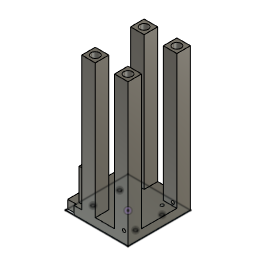
airbee_middle (Autodesk Fusion 360 design; units mm, degrees)
Autodesk Fusion 360 part; units mm, degrees
note: some values were not read from the file. Set by a fixed rule: which sketch regions a step uses.
sketch "Skizze1" plane through (0, 0, 0) normal (0, 0, 1) x (1, 0, 0)
  line L0 (-15.05, 15.05) -> (14.75, 15.05)
  line L1 (14.75, 15.05) -> (14.75, -14.75)
  line L2 (14.75, -14.75) -> (-15.05, -14.75)
  line L3 (-15.05, -14.75) -> (-15.05, 15.05)
  circle A0 centre (-10.41, 6.4) radius 0.75
  circle A1 centre (9.91, 6.4) radius 0.75
  circle A2 centre (-10.41, -6.3) radius 0.75
  circle A3 centre (9.91, -6.3) radius 0.75
  dimension "d1" = 14.75
  dimension "d3" = 14.75
  dimension "d4" = 29.8
  dimension "d5" = 1.5
  dimension "d6" = 1.5
  dimension "d7" = 1.5
  dimension "d8" = 1.5
  dimension "d9" = 20.32
  dimension "d10" = 20.32
  dimension "d11" = 12.7
  dimension "d12" = 12.7
  dimension "d13" = 4.84
  dimension "d14" = 8.65
  dimension "d15" = 4.84
  dimension "d120" = 8.65
  constraint horizontal L0
  constraint vertical L1
  constraint horizontal L2
  constraint vertical L3
  constraint equal L0 L3
  measures "d1" distance of origin L1
  measures "d3" distance of origin L2
  measures "d4" distance of L0.start L2.end
  measures "d5" diameter of A0
  measures "d6" diameter of A1
  measures "d7" diameter of A2
  measures "d8" diameter of A3
  measures "d9" horizontal distance of A0.centre A1.centre
  measures "d10" horizontal distance of A2.centre A3.centre
  measures "d11" vertical distance of A1.centre A3.centre
  measures "d12" vertical distance of A0.centre A2.centre
  measures "d13" distance of L1 A3.centre
  measures "d14" distance of L0 A1.centre
  measures "d15" distance of L1 A1.centre
  measures "d120" distance of L0 A0.centre
extrude "Extrusion1" add sketch "Skizze1" along normal blind 4 contours L0 L1 L2 L3 | A0 | A1 | A2 | A3 makes body 1
sketch "Skizze2" plane through (0, 0, 4) normal (0, 0, 1) x (-1, 0, 0)
  line L0 (15.05, 14.75) -> (-14.75, 14.75)
  line L1 (-14.75, 14.75) -> (-14.75, -15.05)
  line L2 (-14.75, -15.05) -> (15.05, -15.05)
  line L3 (15.05, -15.05) -> (15.05, 14.75)
  circle A0 centre (-3.7, -0.15) radius 9.6
  circle A1 centre (-3.7, -0.15) radius 11.6
  circle A2 centre (-9.91, 6.3) radius 0.75
  line L4 (-14.75, 14.75) -> (15.05, 14.75)
  line L5 (15.05, -15.05) -> (-14.75, -15.05)
  line L6 (15.05, 14.75) -> (11.05, 14.75)
  line L7 (11.05, 14.75) -> (11.05, 13.75)
  line L8 (11.05, 13.75) -> (15.05, 13.75)
  line L9 (15.05, 13.75) -> (15.05, 14.75)
  line L10 (15.05, 14.75) -> (14.05, 14.75)
  line L11 (14.05, 14.75) -> (14.0476, 10.75)
  line L12 (14.0476, 10.75) -> (15.05, 10.75)
  line L13 (15.05, 10.75) -> (15.05, 14.75)
  line L14 (7.35, -15.05) -> (9.05, -15.05)
  line L15 (9.05, -15.05) -> (9.05, 10.35)
  line L16 (9.05, 10.35) -> (7.35, 10.35)
  line L17 (7.35, 10.35) -> (7.35, -15.05)
  line L18 (5.35, -17.05) -> (11.05, -17.05)
  line L19 (11.05, -17.05) -> (11.05, 12.35)
  line L20 (11.05, 12.35) -> (5.35, 12.35)
  line L21 (5.35, 12.35) -> (5.35, -17.05)
  line L22 (5.35, 6.35) -> (11.05, 6.35)
  line L23 (5.35, -11.05) -> (11.05, -11.05)
  line L24 (-14.75, -15.05) -> (-8.2846, -15.05)
  line L25 (-8.2846, -15.05) -> (-8.2846, -8.5846)
  line L26 (-8.2846, -8.5846) -> (-14.75, -8.5846)
  line L27 (-14.75, -8.5846) -> (-14.75, -15.05)
  line L28 (-14.75, 14.75) -> (-8.2846, 14.75)
  line L29 (-8.2846, 14.75) -> (-8.2846, 8.2846)
  line L30 (-8.2846, 8.2846) -> (-14.75, 8.2846)
  line L31 (-14.75, 8.2846) -> (-14.75, 14.75)
  line L32 (7.35, -15.05) -> (0.8846, -15.05)
  line L33 (0.8846, -15.05) -> (0.8846, -8.5846)
  line L34 (0.8846, -8.5846) -> (7.35, -8.5846)
  line L35 (7.35, -8.5846) -> (7.35, -15.05)
  line L36 (0.8846, 14.75) -> (7.35, 14.75)
  line L37 (7.35, 14.75) -> (7.35, 8.2846)
  line L38 (7.35, 8.2846) -> (0.8846, 8.2846)
  line L39 (0.8846, 8.2846) -> (0.8846, 14.75)
  line L40 (9.05, 7.85) -> (11.05, 7.85)
  line L41 (7.35, 8.2846) -> (11.05, 8.2846)
  line L42 (-11.5203, -7.2177) -> (-14.8261, 3.1318)
  line L43 (-11.9705, 6.4686) -> (-11.6289, 6.5777)
  line L44 (-11.6289, 6.5777) -> (-13.2589, 1.4745)
  line L45 (-3.7, -0.15) -> (-14.75, 3.3795)
  line L46 (-3.7, -0.15) -> (-14.75, -3.6795)
  dimension "d18" = 19.2
  dimension "d19" = 2
  dimension "d26" = 14.9
  dimension "d135" = 4
  dimension "d136" = 1
  dimension "d137" = 1
  dimension "d138" = 4
  dimension "d153" = 1.7
  dimension "d154" = 25.4
  dimension "d155" = 2
  dimension "d156" = 4
  dimension "d157" = 4
  dimension "d160" = 6
  dimension "d215" = 11.05
  constraint horizontal L6
  constraint vertical L7
  constraint horizontal L8
  constraint vertical L9
  constraint coincident L0.start L3.end
  constraint horizontal L10
  constraint horizontal L12
  constraint vertical L13
  constraint horizontal L14
  constraint vertical L15
  constraint horizontal L16
  constraint vertical L17
  constraint coincident L5 L14.start
  constraint coincident L21 L22.start
  constraint coincident L19 L22.end
  constraint perpendicular L19 L22
  constraint coincident L21 L23.start
  constraint coincident L19 L23.end
  constraint perpendicular L19 L23
  constraint horizontal L24
  constraint vertical L25
  constraint horizontal L26
  constraint vertical L27
  constraint coincident L1.end L2.start
  constraint horizontal L28
  constraint vertical L29
  constraint horizontal L30
  constraint vertical L31
  constraint coincident L0.end L1.start
  constraint coincident A0 L29.end
  constraint coincident A0 L25.end
  constraint horizontal L32
  constraint vertical L33
  constraint horizontal L34
  constraint vertical L35
  constraint coincident A0 L33.end
  constraint equal L33 L34
  constraint horizontal L36
  constraint vertical L37
  constraint horizontal L38
  constraint vertical L39
  constraint coincident L17 L37.end
  constraint coincident L4 L36.start
  constraint coincident A0 L38.end
  constraint equal L38 L39
  constraint coincident L15 L40.start
  constraint coincident L19 L40.end
  constraint perpendicular L19 L40
  constraint coincident L19 L41.end
  constraint perpendicular L19 L41
  constraint coincident A1 L42.end
  constraint perpendicular L42 L43
  constraint tangent A0 L42
  constraint tangent A0 L44
  constraint perpendicular L42 L46
  constraint perpendicular L44 L45
  constraint coincident A1 L46.end
  constraint coincident L1 L46.end
  constraint coincident A1 L45.end
  constraint coincident L1 L45.end
  constraint coincident A0.centre A1.centre
  constraint equal L25 L26
  constraint coincident L17 L34.end
  constraint equal L29 L30
  measures "d18" diameter of A0
  measures "d26" distance of A0.centre L4
  measures "d135" distance of L0.start L6.end
  measures "d136" distance of L0.start L8.end
  measures "d137" distance of L0.start L10.end
  measures "d138" distance of L0.start L12.end
  measures "d153" distance of L14.start L14.end
  measures "d154" distance of L14.start L16.end
  measures "d156" distance of L16 L22
  measures "d157" distance of L14 L23
  measures "d160" distance of L3 L15
  measures "d215" distance of L1 A0.centre
extrude "Extrusion29" cut sketch "Skizze1" along normal blind 4 contours A0 | A1 | A2 | A3 bodies 1
extrude "Extrusion31" add sketch "Skizze2" along normal blind 10.9 separate body contours L15 L16 L17 L37 L41 | L2 L5 L14 L15 L17 L23 L35 makes body 2 at (-7.35, -9.6615, 11.2667) makes body 3 at (-7.35, 12.3833, 7.6333)
extrude "Extrusion32" add sketch "Skizze2" along normal blind 15 contours L15 L16 L19 L20 L37 L41 | L2 L5 L15 L19 L23 | L15 L19 L40 L41 bodies 1 2 3
extrude "Extrusion34" cut sketch "Skizze2" against normal blind 4 contours L0 L3 L4 L6 L8 L9 L10 L11 L13 | L0 L4 L6 L7 L8 L11 bodies 1
extrude "Extrusion35" add sketch "Skizze2" along normal blind 64 contours L0 A1 L4 L20 L21 L36 L37 L38 L39 | L17 L20 L21 L37 L38 | L0 L1 A1 L4 L28 L29 L30 L31 | A1 L38 L39 | A1 L29 L30 | L2 L5 L17 L21 L23 L32 L35 | L2 A1 L5 L21 L32 L33 L34 | L17 L21 L23 L34 L35 | A1 L33 L34 | L1 L2 A1 L5 L24 L25 L26 L27 | A1 L25 L26 bodies 1
sketch "Skizze9" plane through (0, 0, 68) normal (0, 0, 1) x (-1, 0, 0)
  line L0 (-14.75, 8.2846) -> (-8.2846, 8.2846)
  line L1 (-8.2846, 8.2846) -> (-8.2846, 14.75)
  line L2 (-8.2846, 14.75) -> (-14.75, 14.75)
  line L3 (-14.75, 14.75) -> (-14.75, 8.2846)
  line L4 (-14.75, 14.75) -> (-8.2846, 8.2846)
  line L5 (-14.75, 8.2846) -> (-8.2846, 14.75)
  circle A0 centre (-11.5173, 11.5173) radius 2
  dimension "d225" = 4
  constraint coincident L2.end L3.start
  constraint coincident L0.end L1.start
  constraint coincident L0.start L3.end
  constraint coincident L1.end L2.start
  constraint midpoint L5 A0.centre
  measures "d225" diameter of A0
sketch "Skizze10" plane through (0, 0, 68) normal (0, 0, 1) x (-1, 0, 0)
  line L0 (0.8846, 8.2846) -> (7.35, 8.2846)
  line L1 (7.35, 8.2846) -> (7.35, 14.75)
  line L2 (7.35, 14.75) -> (0.8846, 14.75)
  line L3 (0.8846, 14.75) -> (0.8846, 8.2846)
  line L4 (0.8846, 8.2846) -> (7.35, 14.75)
  line L5 (0.8846, 14.75) -> (7.35, 8.2846)
  circle A0 centre (4.1173, 11.5173) radius 2
  dimension "d226" = 4
  constraint coincident L0.start L3.end
  constraint coincident L1.end L2.start
  constraint coincident L2.end L3.start
  constraint coincident L0.end L1.start
  constraint midpoint L5 A0.centre
  measures "d226" diameter of A0
sketch "Skizze11" plane through (0, 0, 68) normal (0, 0, 1) x (-1, 0, 0)
  line L0 (7.35, -8.5846) -> (0.8846, -8.5846)
  line L1 (0.8846, -8.5846) -> (0.8846, -15.05)
  line L2 (0.8846, -15.05) -> (7.35, -15.05)
  line L3 (7.35, -15.05) -> (7.35, -8.5846)
  line L4 (0.8846, -8.5846) -> (7.35, -15.05)
  line L5 (0.8846, -15.05) -> (7.35, -8.5846)
  circle A0 centre (4.1173, -11.8173) radius 2
  dimension "d227" = 4
  constraint coincident L0.end L1.start
  constraint coincident L2.end L3.start
  constraint coincident L1.end L2.start
  constraint coincident L0.start L3.end
  constraint midpoint L5 A0.centre
  measures "d227" diameter of A0
sketch "Skizze12" plane through (0, 0, 68) normal (0, 0, 1) x (-1, 0, 0)
  line L0 (-14.75, -8.5846) -> (-14.75, -15.05)
  line L1 (-14.75, -15.05) -> (-8.2846, -15.05)
  line L2 (-8.2846, -15.05) -> (-8.2846, -8.5846)
  line L3 (-8.2846, -8.5846) -> (-14.75, -8.5846)
  line L4 (-14.75, -8.5846) -> (-8.2846, -15.05)
  line L5 (-14.75, -15.05) -> (-8.2846, -8.5846)
  circle A0 centre (-11.5173, -11.8173) radius 2
  dimension "d228" = 4
  constraint coincident L0.start L3.end
  constraint coincident L1.end L2.start
  constraint coincident L0.end L1.start
  constraint coincident L2.end L3.start
  constraint midpoint L5 A0.centre
  measures "d228" diameter of A0
extrude "Extrusion36" cut sketch "Skizze10" sketch "Skizze9" sketch "Skizze12" sketch "Skizze11" against normal blind 10 contours L4 L5 A0 | L4 L5 A0 | L4 L5 A0 | L4 L5 A0 of sketch 2 contours L4 L5 A0 | L4 L5 A0 | L4 L5 A0 | L4 L5 A0 of sketch 3 contours L4 L5 A0 | L4 L5 A0 | L4 L5 A0 | L4 L5 A0 of sketch 4 contours L4 L5 A0 | L4 L5 A0 | L4 L5 A0 | L4 L5 A0 bodies 1
sketch "Skizze13" plane through (0, -14.75, 0) normal (0, -1, 0) x (1, 0, 0)
  line L0 (-11.05, 4) -> (-11.05, 0)
  line L1 (-11.05, 0) -> (14.75, 0)
  line L2 (14.75, 0) -> (14.75, 68)
  line L3 (14.75, 68) -> (8.2846, 68)
  line L4 (8.2846, 68) -> (8.2846, 4)
  line L5 (8.2846, 4) -> (-0.8846, 4)
  line L6 (-0.8846, 4) -> (-0.8846, 68)
  line L7 (-0.8846, 68) -> (-7.35, 68)
  line L8 (-7.35, 68) -> (-7.35, 4)
  line L9 (-7.35, 4) -> (-11.05, 4)
  circle A0 centre (12.85, 6) radius 2
  line L10 (14.75, 0) -> (-15.05, 0)
  circle A1 centre (6.35, 6) radius 2
  circle A2 centre (-0.15, 6) radius 2
  circle A3 centre (-6.65, 6) radius 2
  circle A4 centre (-13.15, 6) radius 2
  line L11 (-6.65, 6) -> (-6.65, 5.5)
  circle A5 centre (-6.65, 5.5) radius 1.5
  circle A6 centre (-6.65, 5.5) radius 0.65
  line L12 (12.85, 6) -> (12.85, 5.5)
  circle A7 centre (12.85, 5.5) radius 1.5
  circle A8 centre (12.85, 5.5) radius 0.75
  dimension "d231" = 4
  dimension "d232" = 6
  dimension "d233" = 1.9
  dimension "d236" = -26
  dimension "d237" = 0
  dimension "d240" = 0.5
  dimension "d241" = 3
  dimension "d242" = 1.3
  dimension "d243" = 0.5
  dimension "d244" = 1.5
  constraint coincident A3.centre L11.start
  constraint vertical L11
  constraint coincident L11.end A5.centre
  constraint concentric A5 A6
  constraint coincident A0.centre L12.start
  constraint parallel L2 L12
  constraint coincident L12.end A7.centre
  constraint tangent A0 A7
  constraint concentric A7 A8
  measures "d231" diameter of A0
  measures "d232" distance of A0.centre L10
  measures "d233" distance of L2 A0.centre
  measures "d240" distance of A3.centre L11.end
  measures "d241" diameter of A5
  measures "d242" diameter of A6
  measures "d243" distance of A0.centre L12.end
  measures "d244" diameter of A8
extrude "Extrusion37" cut sketch "Skizze13" against normal blind 29.8 contours A8 bodies 1
equation "d1 = 29.5 mm / 2"
equation "d3 = 29.5 mm / 2"
equation "d13 = ( 30 mm - 0.8 in ) / 2"
equation "d14 = ( 30 mm - 0.5 in ) / 2"
equation "d15 = ( 30 mm - 0.8 in ) / 2"
equation "d26 = ( 29.8 / 2 ) * 1 mm"
equation "d120 = ( 30 mm - 0.5 in ) / 2"
equation "d215 = ( 22.1 / 2 ) * 1 mm"
